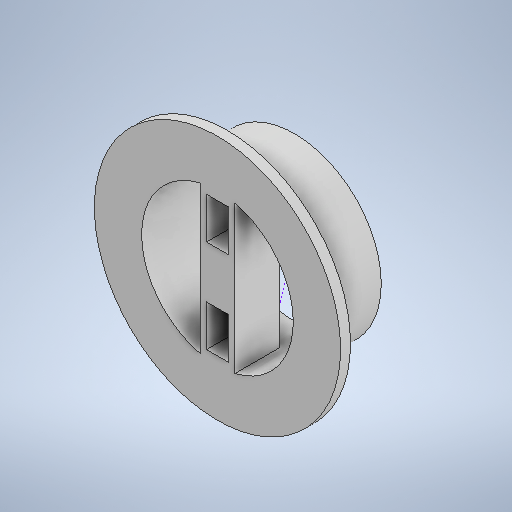
# Autodesk Inventor part: Base_robot_base
Saved by Autodesk Inventor 2025.3 (Build 293356000, 356)
## iProperties
Created: 2025-08-19
Part Number: Base_robot_base
Material: Genérico
Document SubType Name: Modeling
Designer: Rodrigo
Density: 1 g/cm^3
Appearance: Valor por defecto
Author: Rodrigo
## iProperties of the stored document Base_robot_base_3DPrint.ipt
Created: 2025-08-19
Part Number: Base_robot_base_3DPrint
Material: Genérico
Document SubType Name: Modeling
Designer: Rodrigo
Density: 1 g/cm^3
Appearance: Valor por defecto
Author: Rodrigo
Autodesk Inventor part; units mm, degrees
ref_plane "YZ Plane" through (0, 0, 0) normal (1, 0, 0) x (0, 1, 0)
ref_plane "XZ Plane" through (0, 0, 0) normal (0, 1, 0) x (-1, 0, 0)
ref_plane "XY Plane" through (0, 0, 0) normal (0, 0, 1) x (1, 0, 0)
sketch "Boceto1" plane through (0, 0, 0) normal (0, 0, 1) x (1, 0, 0)
  circle A0 centre (0, 0) radius 30.5
  circle A1 centre (0, 0) radius 34.875
  dimension "d0" = 61
  dimension "d1" = 69.75
  constraints: 2 centre point, 2 coincident
  measures "d0" diameter of A0
  measures "d1" diameter of A1
extrude "Extrusión1" add sketch "Boceto1" along normal blind 27
sketch "Boceto2" plane through (0, 0, 27) normal (0, 0, 1) x (1, 0, 0)
  circle A0 centre (0, 0) radius 35.0049
  circle A1 centre (0, 0) radius 30.5
  circle A2 centre (0, 0) radius 49.5
  dimension "d4" = 19
  constraints: 3 centre point, 2 coincident
  measures "d4" radial gap between concentric circles of A1 A2
extrude "Extrusión2" add sketch "Boceto2" along normal blind 4 contours A0 | A2
sketch "Boceto3" plane through (0, 0, 27) normal (0, 0, -1) x (-1, 0, 0)
  point P0 (0, 0)
fillet "Empalme1" radius 7.75 1 edges at (-34.875, 0, 27)
sketch "Boceto4" plane through (0, 0, 0) normal (0, 0, -1) x (-1, 0, 0)
  circle A0 centre (0, 0) radius 31.639
  line L0 (-6.5155, -30.9609) -> (6.5155, -30.9609)
  line L1 (6.5155, -30.9609) -> (6.5155, 30.9609)
  line L2 (6.5155, 30.9609) -> (-6.5155, 30.9609)
  line L3 (-6.5155, 30.9609) -> (-6.5155, -30.9609)
  line L4 (-6.5155, -30.9609) -> (6.5155, 30.9609) construction
  line L5 (6.5155, -30.9609) -> (-6.5155, 30.9609) construction
  constraints: 12 end point, 2 midpoint, 2 parallel, 1 coincident, 1 horizontal, 1 perpendicular, 3 other
sketch "Boceto5" plane through (0, 0, 31) normal (0, 0, 1) x (1, 0, 0)
  line L0 (-7.0125, -31.5254) -> (7.0125, -31.5254)
  line L1 (7.0125, -31.5254) -> (7.0125, 31.5254)
  line L2 (7.0125, 31.5254) -> (-7.0125, 31.5254)
  line L3 (-7.0125, 31.5254) -> (-7.0125, -31.5254)
  line L4 (-7.0125, -31.5254) -> (7.0125, 31.5254) construction
  line L5 (7.0125, -31.5254) -> (-7.0125, 31.5254) construction
  line L6 (-4.4061, -27.0572) -> (4.4061, -27.0572)
  line L7 (4.4061, -27.0572) -> (4.4061, 27.0572)
  line L8 (4.4061, 27.0572) -> (-4.4061, 27.0572)
  line L9 (-4.4061, 27.0572) -> (-4.4061, -27.0572)
  line L10 (-4.4061, -27.0572) -> (4.4061, 27.0572) construction
  line L11 (4.4061, -27.0572) -> (-4.4061, 27.0572) construction
  line L12 (-4.4061, -10.4257) -> (4.4061, -10.4257)
  line L13 (4.4061, -10.4257) -> (4.4061, 10.4257)
  line L14 (4.4061, 10.4257) -> (-4.4061, 10.4257)
  line L15 (-4.4061, 10.4257) -> (-4.4061, -10.4257)
  line L16 (-4.4061, -10.4257) -> (4.4061, 10.4257) construction
  line L17 (4.4061, -10.4257) -> (-4.4061, 10.4257) construction
  point P0 (0, 0)
  constraints: 36 end point, 6 midpoint, 6 parallel, 3 horizontal, 3 perpendicular, 1 point on line
extrude "Extrusión3" add sketch "Boceto5" against normal blind 18 contours L3 L2 L1 L0 | L9 L14 L7 L12
